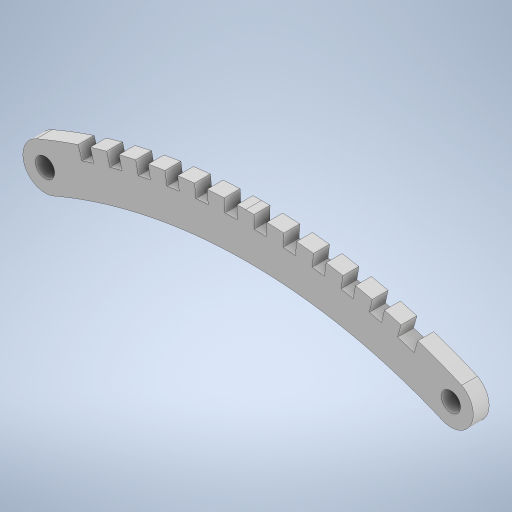
# Autodesk Inventor part: HUDSON-1-73B
Saved by Autodesk Inventor 2024.2 (Build 282272000, 272)
## iProperties
Created: 2024-10-10
Part Number: HUDSON-1-73B
Material: Generic
Document SubType Name: Modeling
Designer: Precisión-10
Density: 1 g/cm^3
Appearance: Default
Author: Precisión-10
Autodesk Inventor part; units mm, degrees
ref_plane "YZ Plane" through (0, 0, 0) normal (1, 0, 0) x (0, 1, 0)
ref_plane "XZ Plane" through (0, 0, 0) normal (0, 1, 0) x (-1, 0, 0)
ref_plane "XY Plane" through (0, 0, 0) normal (0, 0, 1) x (1, 0, 0)
sketch "Sketch1" plane through (0, 0, 0) normal (0, 0, 1) x (1, 0, 0)
  line L0 (0, 0) -> (0, 92) construction
  line L1 (0, 0) -> (-30.243698, 95.920754) construction
  line L2 (0, 0) -> (29.684091, 94.14591) construction
  circle A0 centre (-32, 79.21012) radius 1.5
  circle A1 centre (32, 79.21012) radius 1.5
  circle A2 centre (-32, 79.21012) radius 3.5
  circle A3 centre (32, 79.21012) radius 3.5
  arc A4 (30.625767, 75.991194) -> (-30.625767, 75.991194) centre (0, 4.255133) ccw
  line L3 (-27.979759, 88.740459) -> (0, 0)
  line L4 (-0.976769, 3.783087) -> (0, 0)
  line L5 (0, 82.255133) -> (0, 0)
  line L6 (26.921665, 85.384614) -> (0, 0)
  line L7 (-24.872445, 85.53466) -> (0, 0)
  circle A5 centre (0, 4.255133) radius 85
  circle A6 centre (0, 4.255133) radius 83
  line L8 (-26.784491, 84.949553) -> (-24.872445, 85.53466)
  arc A7 (-24.313944, 83.614015) -> (-26.175937, 83.019467) centre (0, 4.255133) ccw
  line L9 (-22.278402, 86.283621) -> (0, 0)
  line L10 (-20.342287, 86.785076) -> (0, 0)
  line L11 (0, 0) -> (-17.710815, 87.389525)
  line L12 (-24.872445, 85.53466) -> (-22.278402, 86.283621)
  arc A8 (-21.778361, 84.346974) -> (-24.313944, 83.614015) centre (0, 4.255133) ccw
  line L13 (-22.278402, 86.283621) -> (-20.342287, 86.785076)
  arc A9 (-21.778361, 84.346974) -> (-19.88583, 84.837723) centre (0, 4.255133) ccw
  line L14 (-20.342287, 86.785076) -> (-17.710815, 87.389525)
  line L15 (-15.749945, 87.783208) -> (0, 0)
  line L16 (-17.710815, 87.389525) -> (-15.749945, 87.783208)
  line L17 (-13.089089, 88.241297) -> (0, 0)
  line L18 (-15.749945, 87.783208) -> (-13.089089, 88.241297)
  line L19 (-11.109457, 88.526006) -> (0, 0)
  line L20 (-13.089089, 88.241297) -> (-11.109457, 88.526006)
  line L21 (-8.427351, 88.836336) -> (0, 0)
  line L22 (-11.109457, 88.526006) -> (-8.427351, 88.836336)
  line L23 (-6.806993, 94.160062) -> (0, 0)
  line L24 (-8.427351, 88.836336) -> (-6.434774, 89.011217)
  line L25 (-3.816587, 91.008264) -> (0, 0)
  line L26 (-6.434774, 89.011217) -> (-3.739615, 89.17283)
  line L27 (-1.797474, 92.150228) -> (0, 0)
  line L28 (-3.739615, 89.17283) -> (-1.740655, 89.237309)
  line L29 (0, 0) -> (-0.461068, 105.354511) construction
  line L30 (-1.740655, 89.237309) -> (-0.390655, 89.26496)
  line L31 (24.122847, 85.749081) -> (0, 0)
  circle A10 centre (-0.037243, 4.25497) radius 85
  line L32 (26.039941, 85.180731) -> (24.122847, 85.749081)
  arc A11 (25.448304, 83.245393) -> (23.581179, 83.823621) centre (-0.037243, 4.25497) ccw
  line L33 (21.522349, 86.475309) -> (0, 0)
  line L34 (19.581918, 86.959798) -> (0, 0)
  line L35 (0, 0) -> (16.945257, 87.541192)
  line L36 (24.122847, 85.749081) -> (21.522349, 86.475309)
  line L37 (21.522349, 86.475309) -> (19.581918, 86.959798)
  line L38 (19.581918, 86.959798) -> (16.945257, 87.541192)
  line L39 (14.981016, 87.917697) -> (0, 0)
  line L40 (16.945257, 87.541192) -> (14.981016, 87.917697)
  line L41 (12.316253, 88.35248) -> (0, 0)
  line L42 (14.981016, 87.917697) -> (12.316253, 88.35248)
  line L43 (10.334205, 88.619851) -> (0, 0)
  line L44 (12.316253, 88.35248) -> (10.334205, 88.619851)
  line L45 (7.649485, 88.906693) -> (0, 0)
  line L46 (10.334205, 88.619851) -> (7.649485, 88.906693)
  line L47 (5.982593, 94.216033) -> (0, 0)
  line L48 (7.649485, 88.906693) -> (5.655454, 89.064128)
  line L49 (3.019888, 91.038182) -> (0, 0)
  line L50 (5.655454, 89.064128) -> (2.958984, 89.202146)
  line L51 (0.990857, 92.16243) -> (0, 0)
  line L52 (2.958984, 89.202146) -> (0.959536, 89.249126)
  point P0 (-33.374233, 82.429046)
  point P1 (26.175937, 83.019467)
  point P2 (33.374233, 82.429046)
  point P3 (26.777419, 84.927123)
  point P4 (-24.672218, 78.250279)
  point P5 (24.672218, 78.250279)
  point P6 (-25.246691, 83.322223)
  point P7 (-23.049066, 83.990574)
  point P8 (20.83354, -76.087655)
  point P9 (-33.374233, 82.429046)
  point P10 (33.671232, 82.285341)
  point P11 (26.773842, 84.915777)
  point P12 (26.175937, 83.019467)
  point P13 (23.584089, 83.833967)
  point P14 (21.041597, 84.543683)
  point P15 (19.144447, 85.017068)
  point P16 (16.5666, 85.585003)
  point P17 (14.646181, 85.952682)
  point P18 (12.040886, 86.377098)
  point P19 (10.103089, 86.637945)
  point P20 (7.47834, 86.917546)
  point P21 (5.528879, 87.070781)
  point P22 (2.892725, 87.204709)
  point P23 (0.938041, 87.249832)
  point P24 (-0.390608, 89.254236)
  point P25 (-1.70165, 87.237688)
  point P26 (-3.655815, 87.174582)
  point P27 (-6.290566, 87.016409)
  point P28 (-8.238469, 86.845252)
  point P29 (-10.860418, 86.541532)
  point P30 (-12.795626, 86.262889)
  point P31 (-15.396733, 85.814563)
  point P32 (-17.313541, 85.429275)
  point P33 (-26.777419, 84.927123)
  dimension "d37" = 17.5
  dimension "d73" = 170
  dimension "d74" = 166
  dimension "d36" = 92
  dimension "d38" = 17.5
  dimension "d39" = 3
  dimension "d40" = 3
  dimension "d41" = 7
  dimension "d42" = 7
  dimension "d43" = 156
  dimension "d44" = 64
  dimension "d45" = 32
  dimension "d48" = 6.7
  dimension "d78" = 1.99957
  dimension "d79" = 2.7
  dimension "d80" = 2
  dimension "d81" = 2.7
  dimension "d82" = 2
  dimension "d83" = 2.7
  dimension "d84" = 2
  dimension "d85" = 2.7
  dimension "d86" = 2
  dimension "d87" = 2.7
  dimension "d88" = 2
  dimension "d90" = 1.35
  constraints: 48 end point, 18 point on circle, 9 centre point, 3 coincident, 1 equal radius, 1 horizontal alignment, 1 tangent, 1 vertical alignment, 132 other
  measures "d38" angle to the sketch y axis of L2
  measures "d39" diameter of A0
  measures "d40" diameter of A1
  measures "d41" diameter of A2
  measures "d42" diameter of A3
  measures "d43" diameter of A4
  measures "d44" distance of A1.centre A0.centre
  measures "d78" distance of L8.end L8.start
  measures "d79" distance of L12.end L8.end
  measures "d80" distance of L12.end L13.end
  measures "d81" distance of L14.end L13.end
  measures "d82" distance of L16.end L14.end
  measures "d83" distance of L18.end L16.end
  measures "d84" distance of L18.end L20.end
  measures "d85" distance of L20.end L22.end
  measures "d87" distance of L24.end L26.end
  measures "d88" distance of L26.end L28.end
  measures "d90" horizontal distance of L28.end L30.end
sketch "Sketch1 outline for Extrusion3" plane through (0, 0, 0) normal (0, 0, 1) x (1, 0, 0)
  arc A0 (-33.374233, 82.429046) -> (-30.625767, 75.991194) centre (-32, 79.21012) ccw
  arc A1 (-26.777419, 84.927123) -> (-33.374233, 82.429046) centre (0, 4.255133) ccw
  arc A2 (-30.625767, 75.991194) -> (30.625767, 75.991194) centre (0, 4.255133) cw
  line L0 (-26.175937, 83.019467) -> (-26.777419, 84.927123)
  arc A3 (30.625767, 75.991194) -> (33.671232, 82.285341) centre (32, 79.21012) ccw
  arc A4 (-24.313944, 83.614015) -> (-26.175937, 83.019467) centre (0, 4.255133) ccw
  arc A5 (33.671232, 82.285341) -> (26.773842, 84.915777) centre (-0.037243, 4.25497) ccw
  line L1 (-24.872445, 85.53466) -> (-24.313944, 83.614015)
  line L2 (26.773842, 84.915777) -> (26.175937, 83.019467)
  line L3 (-22.278402, 86.283621) -> (-24.872445, 85.53466)
  arc A6 (26.175937, 83.019467) -> (23.584089, 83.833967) centre (0, 4.255133) ccw
  line L4 (-21.778361, 84.346974) -> (-22.278402, 86.283621)
  line L5 (23.584089, 83.833967) -> (24.122847, 85.749081)
  arc A7 (-19.88583, 84.837723) -> (-21.778361, 84.346974) centre (0, 4.255133) ccw
  line L6 (24.122847, 85.749081) -> (21.522349, 86.475309)
  line L7 (-20.342287, 86.785076) -> (-19.88583, 84.837723)
  line L8 (21.522349, 86.475309) -> (21.041597, 84.543683)
  line L9 (-17.710815, 87.389525) -> (-20.342287, 86.785076)
  arc A8 (21.041597, 84.543683) -> (19.144447, 85.017068) centre (0, 4.255133) ccw
  line L10 (-17.313541, 85.429275) -> (-17.710815, 87.389525)
  line L11 (19.144447, 85.017068) -> (19.581918, 86.959798)
  arc A9 (-15.396733, 85.814563) -> (-17.313541, 85.429275) centre (0, 4.255133) ccw
  line L12 (19.581918, 86.959798) -> (16.945257, 87.541192)
  line L13 (-15.749945, 87.783208) -> (-15.396733, 85.814563)
  line L14 (16.945257, 87.541192) -> (16.5666, 85.585003)
  line L15 (-13.089089, 88.241297) -> (-15.749945, 87.783208)
  arc A10 (16.5666, 85.585003) -> (14.646181, 85.952682) centre (0, 4.255133) ccw
  line L16 (-12.795626, 86.262889) -> (-13.089089, 88.241297)
  line L17 (14.646181, 85.952682) -> (14.981016, 87.917697)
  arc A11 (-10.860418, 86.541532) -> (-12.795626, 86.262889) centre (0, 4.255133) ccw
  line L18 (14.981016, 87.917697) -> (12.316253, 88.35248)
  line L19 (-11.109457, 88.526006) -> (-10.860418, 86.541532)
  line L20 (12.316253, 88.35248) -> (12.040886, 86.377098)
  line L21 (-8.427351, 88.836336) -> (-11.109457, 88.526006)
  arc A12 (12.040886, 86.377098) -> (10.103089, 86.637945) centre (0, 4.255133) ccw
  line L22 (-8.238469, 86.845252) -> (-8.427351, 88.836336)
  line L23 (10.103089, 86.637945) -> (10.334205, 88.619851)
  arc A13 (-6.290566, 87.016409) -> (-8.238469, 86.845252) centre (0, 4.255133) ccw
  line L24 (10.334205, 88.619851) -> (7.649485, 88.906693)
  line L25 (-6.434774, 89.011217) -> (-6.290566, 87.016409)
  line L26 (7.649485, 88.906693) -> (7.47834, 86.917546)
  line L27 (-3.739615, 89.17283) -> (-6.434774, 89.011217)
  arc A14 (7.47834, 86.917546) -> (5.528879, 87.070781) centre (0, 4.255133) ccw
  line L28 (-3.655815, 87.174582) -> (-3.739615, 89.17283)
  line L29 (5.528879, 87.070781) -> (5.655454, 89.064128)
  arc A15 (-1.70165, 87.237688) -> (-3.655815, 87.174582) centre (0, 4.255133) ccw
  line L30 (5.655454, 89.064128) -> (2.958984, 89.202146)
  line L31 (-1.740655, 89.237309) -> (-1.70165, 87.237688)
  line L32 (2.958984, 89.202146) -> (2.892725, 87.204709)
  arc A16 (-0.390608, 89.254236) -> (-1.740655, 89.237309) centre (0, 4.255133) ccw
  arc A17 (2.892725, 87.204709) -> (0.938041, 87.249832) centre (0, 4.255133) ccw
  arc A18 (0.959536, 89.249126) -> (-0.390608, 89.254236) centre (-0.037243, 4.25497) ccw
  line L33 (0.938041, 87.249832) -> (0.959536, 89.249126)
  circle A19 centre (-32, 79.21012) radius 1.5
  circle A20 centre (32, 79.21012) radius 1.5
extrude "Extrusion3" add sketch "Sketch1 outline for Extrusion3" along normal blind 2.5
body "Solid3"
